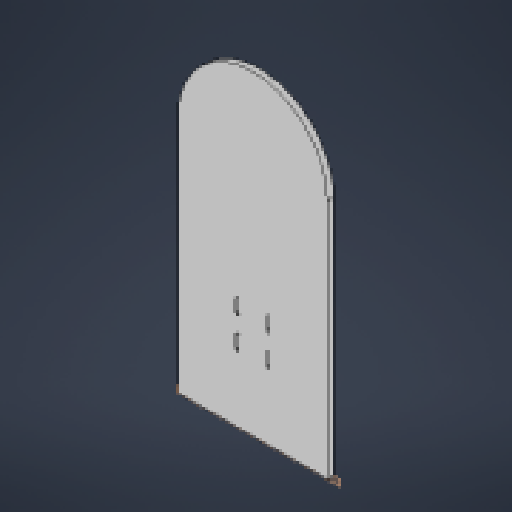
# Autodesk Inventor part: SideBoard
Saved by Autodesk Inventor 2024 (Build 280153000, 153)
## iProperties
Created: 2023-10-21
Part Number: SideBoard
Material: Generic
Document SubType Name: Modeling
Designer: range
Density: 1 g/cm^3
Appearance: Default
Author: range
Autodesk Inventor part; units mm, degrees
ref_plane "YZ Plane" through (0, 0, 0) normal (1, 0, 0) x (0, 1, 0)
ref_plane "XZ Plane" through (0, 0, 0) normal (0, 1, 0) x (-1, 0, 0)
ref_plane "XY Plane" through (0, 0, 0) normal (0, 0, 1) x (1, 0, 0)
ref_plane "Work Plane1" through (0, 0, 0) normal (0, 0, 1) x (1, 0, 0)
sketch "Sketch1" plane through (0, 0, 0) normal (0, 0, 1) x (1, 0, 0)
  line L0 (0, 0) -> (150, 0) projected
  line L1 (150, 0) -> (150, 6.35) projected
  line L2 (0, 6.35) -> (150, 6.35) projected
  line L3 (0, 0) -> (0, 6.35) projected
  line L4 (-41.185, 45.466) -> (-34.327, 45.466) projected
  line L5 (0, 6.35) -> (0, 45.466)
  line L6 (150, 6.35) -> (150, 45.466)
  line L7 (0, 45.466) -> (150, 45.466) construction
  line L8 (75, 45.466) -> (75, 96.266) construction
  line L9 (75, 96.266) -> (75, 248.666) construction
  line L10 (59.506, 80.772) -> (90.494, 80.772)
  line L11 (90.494, 80.772) -> (90.494, 111.76)
  line L12 (90.494, 111.76) -> (59.506, 111.76)
  line L13 (59.506, 111.76) -> (59.506, 80.772)
  line L14 (59.506, 80.772) -> (90.494, 111.76) construction
  line L15 (90.494, 80.772) -> (59.506, 111.76) construction
  line L16 (90.494, 118.11) -> (90.494, 105.41) construction
  line L17 (88.994, 118.11) -> (88.994, 105.41)
  line L18 (91.994, 105.41) -> (91.994, 118.11)
  arc A0 (91.994, 118.11) -> (88.994, 118.11) centre (90.494, 118.11) ccw
  arc A1 (88.994, 105.41) -> (91.994, 105.41) centre (90.494, 105.41) ccw
  line L19 (90.494, 74.422) -> (90.494, 87.122) construction
  line L20 (91.994, 74.422) -> (91.994, 87.122)
  line L21 (88.994, 87.122) -> (88.994, 74.422)
  arc A2 (88.994, 74.422) -> (91.994, 74.422) centre (90.494, 74.422) ccw
  arc A3 (91.994, 87.122) -> (88.994, 87.122) centre (90.494, 87.122) ccw
  line L22 (59.506, 105.41) -> (59.506, 118.11) construction
  line L23 (61.006, 105.41) -> (61.006, 118.11)
  line L24 (58.006, 118.11) -> (58.006, 105.41)
  arc A4 (58.006, 105.41) -> (61.006, 105.41) centre (59.506, 105.41) ccw
  arc A5 (61.006, 118.11) -> (58.006, 118.11) centre (59.506, 118.11) ccw
  line L25 (59.506, 74.422) -> (59.506, 87.122) construction
  line L26 (61.006, 74.422) -> (61.006, 87.122)
  line L27 (58.006, 87.122) -> (58.006, 74.422)
  arc A6 (58.006, 74.422) -> (61.006, 74.422) centre (59.506, 74.422) ccw
  arc A7 (61.006, 87.122) -> (58.006, 87.122) centre (59.506, 87.122) ccw
  line L28 (0, 45.466) -> (0, 248.666)
  line L29 (150, 45.466) -> (150, 248.666)
  circle A8 centre (75, 248.666) radius 75
  circle A9 centre (75, 316.966) radius 5.1943 projected
  circle A10 centre (6.7, 248.666) radius 5.1943 projected
  circle A11 centre (75, 180.366) radius 5.1943 projected
  circle A12 centre (143.3, 248.666) radius 5.1943 projected
  circle A13 centre (75, 248.666) radius 74.3 projected
  circle A14 centre (75, 248.666) radius 62.3 projected
  circle A15 centre (143.3, 248.666) radius 2.5
  circle A16 centre (75, 316.966) radius 2.5
  circle A17 centre (6.7, 248.666) radius 2.5
  circle A18 centre (75, 180.366) radius 2.5
  circle A19 centre (75, 96.266) radius 11.493 construction
  line L30 (75, 89.916) -> (75, 102.616) construction
  line L31 (63.507, 89.916) -> (63.507, 102.616)
  line L32 (86.493, 102.616) -> (86.493, 89.916)
  arc A20 (63.507, 89.916) -> (86.493, 89.916) centre (75, 89.916) ccw
  arc A21 (86.493, 102.616) -> (63.507, 102.616) centre (75, 102.616) ccw
  dimension "d0" = 50.8
  dimension "d1" = 152.4
  dimension "d2" = 30.988
  dimension "d3" = 30.988
  dimension "d4" = 6.35
  dimension "d5" = 3
  dimension "d6" = 6.35
  dimension "d7" = 3
  dimension "d8" = 6.35
  dimension "d9" = 3
  dimension "d10" = 6.35
  dimension "d11" = 3
  dimension "d14" = 5
  dimension "d17" = 360
  dimension "d19" = 6.35
  constraints: 66 end point, 21 tangent, 20 point on circle, 15 centre point, 8 midpoint, 8 parallel, 7 point on line, 6 vertical, 3 coincident, 2 horizontal, 1 perpendicular, 14 other
  measures "d0" distance of L8.start L8.end
  measures "d1" distance of L8.end L9.end
  measures "d2" distance of L12.end L11.end
  measures "d3" distance of L11.end L10.end
  measures "d4" distance of L11.end L16.end
  measures "d5" diameter of A1
  measures "d6" distance of L10.end L19.end
  measures "d7" diameter of A3
  measures "d8" distance of L12.end L22.end
  measures "d9" diameter of A5
  measures "d10" distance of L10.start L25.end
  measures "d11" diameter of A7
  measures "d14" diameter of A15
  measures "d19" distance of A19.centre L30.end
extrude "Extrusion1" add sketch "Sketch1" along normal blind 6.35 contours L3 L2 L1 L0 | L5 L28 A8 L29 L6 L2 | A8 | L26 A7 L13 A4 L23 L12 A21 L31 A20 L10 | A20 L32 A21 L12 L17 A1 L11 A3 L21 L10 | A9 | A10 | A11 | A12 | A13
body "Solid1"
